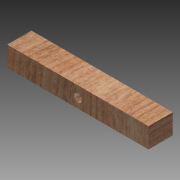
# Autodesk Inventor part: CNC-X-axis- platform mover
Saved by Autodesk Inventor 2015 (Build 190159000, 159)
## iProperties
Created: 2015-03-30
Part Number: CNC-X-axis- platform mover
Material: Generic
Document SubType Name: Modeling
Designer: Bangladesh
Density: 1 g/cm^3
Appearance: Default
Author: Bangladesh
Autodesk Inventor part; units mm, degrees
ref_plane "YZ Plane" through (0, 0, 0) normal (1, 0, 0) x (0, 1, 0)
ref_plane "XZ Plane" through (0, 0, 0) normal (0, 1, 0) x (-1, 0, 0)
ref_plane "XY Plane" through (0, 0, 0) normal (0, 0, 1) x (1, 0, 0)
sketch "Sketch1" plane through (0, 0, 0) normal (0, 0, 1) x (1, 0, 0)
  line L0 (-111.1, 15.875) -> (111.1, 15.875)
  line L1 (111.1, 15.875) -> (111.1, -15.875)
  line L2 (111.1, -15.875) -> (-111.1, -15.875)
  line L3 (-111.1, -15.875) -> (-111.1, 15.875)
  line L4 (-111.1, 15.875) -> (111.1, -15.875) construction
  line L5 (111.1, 15.875) -> (-111.1, -15.875) construction
  point P0 (0, 0)
  dimension "d0" = 31.75
  dimension "d1" = 222.2
  constraints: 12 end point, 2 midpoint, 2 parallel, 1 horizontal, 1 perpendicular
  measures "d0" distance of L0.end L1.end
  measures "d1" distance of L0.start L0.end
extrude "Extrusion1" add sketch "Sketch1" along normal mid plane 38.1
sketch "Sketch2" plane through (0, 0, 19.05) normal (0, 0, 1) x (1, 0, 0)
  circle A0 centre (0, -1.5469) radius 6.619
  line L0 (-1.3396, -8.0289) -> (-6.2834, -3.6278)
  line L1 (-6.2834, -3.6278) -> (-4.9438, 2.8543)
  line L2 (-4.9438, 2.8543) -> (1.3396, 4.9352)
  line L3 (1.3396, 4.9352) -> (6.2834, 0.534)
  line L4 (6.2834, 0.534) -> (4.9438, -5.948)
  line L5 (4.9438, -5.948) -> (-1.3396, -8.0289)
  line L6 (111.1, 15.875) -> (-111.1, 15.875) projected
  dimension "d10" = 17.4219
  constraints: 12 end point, 1 coincident, 16 other
  measures "d10" distance from line of L6 point (0, -1.547)
extrude "Extrusion2" cut sketch "Sketch2" against normal blind 82.55 contours L4 L5 L0 L1 L2 L3
body "Solid1"
